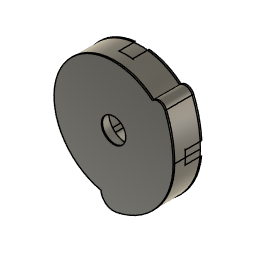
Servo Cams v5 (Autodesk Fusion 360 design; units mm, degrees)
Autodesk Fusion 360 part; units mm, degrees
sketch "Sketch1" plane through (0, 0, 0) normal (0, 1, 0) x (1, 0, 0)
  circle A0 centre (0, 0) radius 11.7
  line L0 (0, 0) -> (0, 11.7)
  line L1 (0, 0) -> (11.7, 0) construction
  line L2 (0, 0) -> (0, 11.25)
  circle A1 centre (0, 11.25) radius 2.5
  circle A2 centre (2.2784, 0) radius 13.9784 construction
  line L3 (0, 11.25) -> (0, 13.75) construction
  line L4 (0, 0) -> (-11.7, 0) construction
  arc A3 (-0.4962, 13.7003) -> (-11.7, 0) centre (2.2784, 0) ccw
  line L5 (0, 0) -> (0, 5.85)
  line L6 (0, 0) -> (-8.6948, -7.8288) construction
  circle A4 centre (-8.6948, -7.8288) radius 1.5
  circle A5 centre (10.9122, 0) radius 22.6122
  dimension "d1" = 23.4
  dimension "d2" = 90
  dimension "d3" = 11.25
  dimension "d4" = 5
  dimension "d56" = 27.9568
  dimension "d62" = 132
  dimension "d63" = 3
  constraint coincident A0.centre L0.start
  constraint horizontal L1
  constraint coincident A0 L0.end
  constraint parallel L0 L2
  constraint coincident L2.end A1.centre
  constraint coincident A1 L3.end
  constraint parallel L0 L3
  constraint coincident A0 L4.end
  constraint perpendicular L2 L4
  constraint coincident A2 L4.end
  constraint tangent A1 A2
  constraint tangent A0 A2
  constraint coincident A1 A3.start
  constraint coincident A2.centre A3.centre
  constraint midpoint L0 L5.end
  constraint coincident A0 L6.end
  constraint coincident L6.end A4.centre
  constraint coincident L4.end A5
  constraint tangent A4 A5
  constraint tangent A0 A5
  measures "d1" diameter of A0
  measures "d2" angle of L0 L1
  measures "d3" distance of A0.centre L2.end
  measures "d4" diameter of A1
  measures "d56" diameter of A2
  measures "d62" angle of L5 L6
  measures "d63" diameter of A4
extrude "Extrude1" add sketch "Sketch1" against normal blind 5.35 contours A0 A1 A4 | A0 L0 L2 A1 | A0 A1 | A0 A4 | A0 A4 | A0 L0 L2 A1 | A0 A1 A3 | A0 A4 A5 makes body 1
move_body "Move2" bodies 1 to x (-1, 0, 0) y (0, -1, 0) z (0, 0, 1) at (0, 0, 0)
copy_body "CopyPasteBodies1" bodies 1 makes body 2
sketch "Servo_Cam_Savox" plane through (0, 0, 0) normal (0, 1, 0) x (1, 0, 0)
  arc A0 (11.7, 0) -> (0.4962, 13.7003) centre (-2.2784, 0) ccw
  arc A1 (0.4962, 13.7003) -> (-2.4934, 11.4312) centre (0, 11.25) ccw
  arc A2 (-2.4934, 11.4312) -> (7.6217, -8.8769) centre (0, 0) ccw
  line L0 (-10.4, -2) -> (10.4, -2)
  arc A3 (10.4, -2) -> (10.4, 2) centre (10.4, 0) ccw construction
  line L1 (10.4, 2) -> (-10.4, 2)
  arc A4 (-10.4, 2) -> (-10.4, -2) centre (-10.4, 0) ccw construction
  line L2 (-12.4, 0) -> (12.4, 0) construction
  line L3 (2, -10.4) -> (2, 10.4)
  arc A5 (2, 10.4) -> (-2, 10.4) centre (0, 10.4) ccw construction
  line L4 (-2, 10.4) -> (-2, -10.4)
  arc A6 (-2, -10.4) -> (2, -10.4) centre (0, -10.4) ccw construction
  line L5 (0, -12.4) -> (0, 12.4) construction
  circle A7 centre (0, 0) radius 3.5 construction
  circle A8 centre (5.45, -5.45) radius 3.45
  circle A9 centre (-5.45, -5.45) radius 3.45
  circle A10 centre (-5.45, 5.45) radius 3.45
  circle A11 centre (5.45, 5.45) radius 3.45
  circle A12 centre (0, 0) radius 3.6
  arc A13 (-10.4, 2.05) -> (-10.4, -2.05) centre (-10.4, 0) ccw
  line L6 (-10.4, -2.05) -> (10.4, -2.05)
  arc A14 (10.4, -2.05) -> (10.4, 2.05) centre (10.4, 0) ccw
  line L7 (10.4, 2.05) -> (-10.4, 2.05)
  arc A15 (-2.05, -10.4) -> (2.05, -10.4) centre (0, -10.4) ccw
  line L8 (2.05, -10.4) -> (2.05, 10.4)
  arc A16 (2.05, 10.4) -> (-2.05, 10.4) centre (0, 10.4) ccw
  line L9 (-2.05, 10.4) -> (-2.05, -10.4)
  circle A17 centre (-5.55, -5.55) radius 3.5 construction
  circle A18 centre (-5.55, 5.55) radius 3.5 construction
  circle A19 centre (5.55, 5.55) radius 3.5 construction
  circle A20 centre (5.55, -5.55) radius 3.5 construction
  circle A21 centre (0, 0) radius 1
  circle A22 centre (0, 0) radius 2.4
  line L10 (-10.4, 0) -> (-10.4, -2.9358)
  line L11 (-10.4, -2.9358) -> (-10.4, 2.7529)
  line L12 (0, -10.4) -> (2.9295, -10.4)
  line L13 (2.9295, -10.4) -> (-3.2418, -10.4)
  line L14 (10.4, 0) -> (10.4, -3.6257)
  line L15 (10.4, -3.6257) -> (10.4, 2.9985)
  line L16 (0, 10.4) -> (2.8729, 10.4)
  line L17 (2.8729, 10.4) -> (-3.6947, 10.4)
  arc A23 (7.6217, -8.8769) -> (10.0879, -8.3851) centre (8.6948, -7.8288) ccw
  arc A24 (10.0879, -8.3851) -> (11.7, 0) centre (-10.9122, 0) ccw
  dimension "d7" = 4
  dimension "d8" = 4
  dimension "d9" = 7
  dimension "d10" = 3.45
  dimension "d11" = 3.45
  dimension "d12" = 3.45
  dimension "d13" = 3.45
  dimension "d32" = 0.1
  dimension "d33" = 0.05
  dimension "d34" = 0.05
  dimension "d35" = 7
  dimension "d36" = 7
  dimension "d37" = 7
  dimension "d38" = 7
  dimension "d39" = 2
  dimension "d51" = 24.8
  dimension "d52" = 4.8
  dimension "d53" = 24.8
  constraint tangent L0 A3
  constraint tangent A3 L1
  constraint parallel L0 L1
  constraint tangent L1 A4
  constraint tangent L0 A4
  constraint midpoint A4 L2.start
  constraint midpoint A3 L2.end
  constraint horizontal L2
  constraint tangent L3 A5
  constraint tangent A5 L4
  constraint parallel L3 L4
  constraint tangent L4 A6
  constraint tangent L3 A6
  constraint midpoint A6 L5.start
  constraint midpoint A5 L5.end
  constraint perpendicular L1 L5
  constraint midpoint L5 A2.centre
  constraint midpoint L2 A2.centre
  constraint coincident A2.centre A7.centre
  constraint concentric A2 A7
  constraint tangent L0 A8
  constraint tangent L3 A8
  constraint tangent L0 A9
  constraint tangent L4 A9
  constraint tangent L4 A10
  constraint tangent L1 A10
  constraint tangent L3 A11
  constraint tangent L1 A11
  constraint tangent L8 A20
  constraint tangent L6 A20
  constraint tangent L6 A17
  constraint tangent L9 A17
  constraint tangent L7 A18
  constraint tangent L9 A18
  constraint tangent L8 A19
  constraint tangent L7 A19
  constraint coincident A4.centre A13.centre
  constraint perpendicular L0 L10
  constraint perpendicular L7 L11
  constraint coincident A6.centre A15.centre
  constraint perpendicular L3 L12
  constraint parallel L12 L13
  constraint coincident A3.centre A14.centre
  constraint perpendicular L0 L14
  constraint perpendicular L2 L15
  constraint coincident A5.centre A16.centre
  constraint perpendicular L8 L16
  constraint perpendicular L9 L17
  measures "d7" diameter of A3
  measures "d8" diameter of A5
  measures "d9" diameter of A7
  measures "d10" radius of A8
  measures "d11" radius of A9
  measures "d12" radius of A10
  measures "d13" radius of A11
  measures "d35" diameter of A17
  measures "d36" diameter of A18
  measures "d37" diameter of A19
  measures "d38" diameter of A20
  measures "d39" diameter of A21
  measures "d51" distance of L5.start L5.end
  measures "d52" diameter of A22
  measures "d53" distance of L2.start L2.end
extrude "Extrude2" cut sketch "Servo_Cam_Savox" against normal blind 1.8 from surface at 5.35 contours L0 L1 A12 L14 L15 | L1 A11 A12 L7 | A11 A12 L7 L8 | L0 A8 A12 L6 | A8 A12 L6 L8 | L0 L1 A12 L8 A22 | L1 A12 L7 L8 | L3 A11 A12 L8 | A12 L7 L8 | L0 A12 L6 L8 | L3 A8 A12 L8 | A12 L6 L8 | L0 L1 A12 L10 L11 | L1 L3 L8 A22 | L1 L3 L7 L8 | L3 L4 A12 L16 L17 | L3 A12 L7 L8 | L3 L4 A12 L12 L13 | L0 L3 L6 L8 | L0 L3 L8 A22 | L3 A12 L6 L8 | L1 A10 A12 L7 | A10 A12 L7 L9 | L1 L3 A22 | L1 L3 L7 A22 | L8 A22 | L3 L8 A22 | L3 L4 A12 L7 A22 | L3 L4 A12 L6 A22 | L0 L3 L6 A22 | L0 L3 A22 | L0 A9 A12 L6 | A9 A12 L6 L9 | L4 A10 A12 L9 | L1 A12 L7 L9 | L0 L1 A12 L9 A22 | A12 L7 L9 | L0 L1 L3 L4 A22 | L1 L7 A22 | L4 A12 L7 L9 | L7 A22 | L4 A12 L6 L9 | L4 A9 A12 L9 | L0 L6 A22 | L6 A22 | L0 A12 L6 L9 | A12 L6 L9 | L1 L4 L7 L9 | L1 L4 L9 A22 | L1 L4 A22 | L1 L4 L7 A22 | L0 L4 L6 L9 | L0 L4 L6 A22 | L0 L4 A22 | L0 L4 L9 A22 | L4 L9 A22 | L9 A22 | A21 bodies 1
extrude "Extrude3" cut sketch "Servo_Cam_Savox" against normal blind 4.2 from surface at 5.35 contours L0 L1 A12 L8 A22 | L1 A12 L7 L8 | A12 L7 L8 | L0 A12 L6 L8 | A12 L6 L8 | L1 L3 L8 A22 | L1 L3 L7 L8 | L3 A12 L7 L8 | L0 L3 L6 L8 | L0 L3 L8 A22 | L3 A12 L6 L8 | L1 L3 A22 | L1 L3 L7 A22 | L8 A22 | L3 L8 A22 | L3 L4 A12 L7 A22 | L3 L4 A12 L6 A22 | L0 L3 L6 A22 | L0 L3 A22 | L1 A12 L7 L9 | L0 L1 A12 L9 A22 | A12 L7 L9 | L0 L1 L3 L4 A22 | L1 L7 A22 | L4 A12 L7 L9 | L7 A22 | L4 A12 L6 L9 | L0 L6 A22 | L6 A22 | L0 A12 L6 L9 | A12 L6 L9 | L1 L4 L7 L9 | L1 L4 L9 A22 | L1 L4 A22 | L1 L4 L7 A22 | L0 L4 L6 L9 | L0 L4 L6 A22 | L0 L4 A22 | L0 L4 L9 A22 | L4 L9 A22 | L9 A22 | A21 bodies 1
extrude "Extrude6" cut sketch "Servo_Cam_Savox" along normal blind 21.2848 contours L8 A22 | L3 L8 A22 | L0 L1 L3 L4 A22 | L1 L7 A22 | L7 A22 | L0 L6 A22 | L6 A22 | L4 L9 A22 | L9 A22 | A21 bodies 1
sketch "Servo_Cam_DS041MG" plane through (0, 0, 0) normal (0, 1, 0) x (1, 0, 0)
  arc A0 (11.7, 0) -> (0.4962, 13.7003) centre (-2.2784, 0) ccw
  arc A1 (-2.4934, 11.4312) -> (7.6217, -8.8769) centre (0, 0) ccw
  arc A2 (0.4962, 13.7003) -> (-2.4934, 11.4312) centre (0, 11.25) ccw
  circle A3 centre (0, 0) radius 3.95 construction
  line L0 (9.45, 2.5) -> (-9.45, 2.5) construction
  arc A4 (-9.45, 2.5) -> (-9.45, -2.5) centre (-9.45, 0) ccw construction
  line L1 (-9.45, -2.5) -> (9.45, -2.5) construction
  arc A5 (9.45, -2.5) -> (9.45, 2.5) centre (9.45, 0) ccw construction
  line L2 (11.95, 0) -> (-11.95, 0) construction
  line L3 (2.5, -9.45) -> (2.5, 9.45) construction
  arc A6 (2.5, 9.45) -> (-2.5, 9.45) centre (0, 9.45) ccw construction
  line L4 (-2.5, 9.45) -> (-2.5, -9.45) construction
  arc A7 (-2.5, -9.45) -> (2.5, -9.45) centre (0, -9.45) ccw construction
  line L5 (0, -11.95) -> (0, 11.95) construction
  line L6 (9.45, 2.55) -> (-9.45, 2.55)
  arc A8 (-9.45, 2.55) -> (-9.45, -2.55) centre (-9.45, 0) ccw
  line L7 (-9.45, -2.55) -> (9.45, -2.55)
  arc A9 (9.45, -2.55) -> (9.45, 2.55) centre (9.45, 0) ccw
  line L8 (-2.55, 9.45) -> (-2.55, -9.45)
  arc A10 (-2.55, -9.45) -> (2.55, -9.45) centre (0, -9.45) ccw
  line L9 (2.55, -9.45) -> (2.55, 9.45)
  arc A11 (2.55, 9.45) -> (-2.55, 9.45) centre (0, 9.45) ccw
  circle A12 centre (0, 0) radius 4
  circle A13 centre (0, 0) radius 1.3
  circle A14 centre (0, 0) radius 2.5
  line L10 (0, 9.45) -> (0, 6.95)
  line L11 (3.7291, 6.95) -> (-3.9575, 6.95)
  arc A15 (7.6217, -8.8769) -> (10.0879, -8.3851) centre (8.6948, -7.8288) ccw
  arc A16 (10.0879, -8.3851) -> (11.7, 0) centre (-10.9122, 0) ccw
  dimension "d20" = 7.9
  dimension "d21" = 5
  dimension "d22" = 5
  dimension "d23" = 0.05
  dimension "d24" = 0.05
  dimension "d25" = 0.05
  dimension "d42" = 2.6
  dimension "d45" = 23.9
  dimension "d46" = 23.9
  dimension "d47" = 5
  dimension "d48" = 2.5
  constraint concentric A1 A3
  constraint tangent L0 A4
  constraint tangent A4 L1
  constraint parallel L0 L1
  constraint tangent L1 A5
  constraint tangent L0 A5
  constraint midpoint A5 L2.start
  constraint midpoint A4 L2.end
  constraint horizontal L2
  constraint tangent L3 A6
  constraint tangent A6 L4
  constraint parallel L3 L4
  constraint tangent L4 A7
  constraint tangent L3 A7
  constraint midpoint A7 L5.start
  constraint midpoint A6 L5.end
  constraint vertical L5
  constraint midpoint L2 A1.centre
  constraint midpoint L5 A1.centre
  constraint coincident A1.centre A3.centre
  constraint coincident A6.centre A11.centre
  constraint parallel L5 L10
  constraint perpendicular L8 L11
  measures "d20" diameter of A3
  measures "d21" diameter of A4
  measures "d22" diameter of A6
  measures "d42" diameter of A13
  measures "d45" distance of L5.start L5.end
  measures "d46" distance of L2.start L2.end
  measures "d47" diameter of A14
  measures "d48" distance of A6.centre L10.end
extrude "Extrude4" cut sketch "Servo_Cam_DS041MG" against normal blind 2 from surface at 5.35 contours A0 L6 L7 A9 A12 A16 | A0 A9 A16 | L6 L7 L9 A12 | L6 L9 A12 | L7 L9 A12 | A1 L6 A8 L7 A12 | A1 A8 | L6 L7 L8 L9 | L6 L8 L9 A12 | L8 L9 A12 L11 | L7 L8 L9 A12 | A1 L8 A10 L9 A12 | A1 A10 | L6 L7 L8 A12 | L6 L8 A12 | L7 L8 A12 | A13 | A14 bodies 2
extrude "Extrude5" cut sketch "Servo_Cam_DS041MG" against normal blind 4.1 from surface at 5.35 contours L6 L7 L9 A12 | L6 L9 A12 | L7 L9 A12 | L6 L7 L8 L9 | L6 L8 L9 A12 | L7 L8 L9 A12 | L6 L7 L8 A12 | L6 L8 A12 | L7 L8 A12 | A13 | A14 bodies 2
extrude "Extrude7" cut sketch "Servo_Cam_DS041MG" along normal blind 5.372 contours A13 | A14 bodies 2
extrude "Extrude8" cut 1 faces at (0.7217, 0, -8.7686) along direction (0, 1, 0) blind 1.25 on bodies 2 bodies 2
extrude "Extrude9" cut 1 faces at (0.7143, 0, -8.7361) along direction (0, 1, 0) blind 0.95 on bodies 1 bodies 1
extrude "Extrude10" add 1 faces at (5.3308, 5.35, -5.433) along direction (0, 1, 0) blind 0.95 on bodies 1 bodies 1
extrude "Extrude11" add 3 faces at (0.8209, 5.35, -10.5171) (-4.2446, 5.35, 7.1328) (6.7178, 5.35, 4.659) along direction (0, 1, 0) blind 1.25 on bodies 2 bodies 2
equation "d10 = ( 6.9 / 2 ) * 1 mm"
equation "d58 = 5.35 mm - 4.4 mm"
equation "d60 = 5.35 mm - 4.1 mm"
named bodies: "Servo_Cam_Savox", "Servo_Cam_DS041MG"
